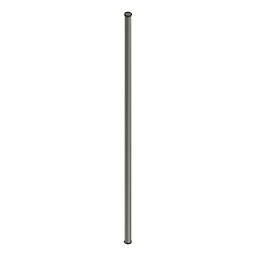
Rainfall sensor mid september v4 (Autodesk Fusion 360 archive; units mm, degrees)
design "graphite rod"
Autodesk Fusion 360 part; units mm, degrees
sketch "Sketch1" plane through (0, 0, 0) normal (0, 0, 1) x (1, 0, 0)
  circle A0 centre (0, 0) radius 1
  dimension "d1" = 2
  constraint coincident A0.centre origin
  measures "d1" diameter of A0
extrude "Extrude1" add sketch "Sketch1" along normal blind 80

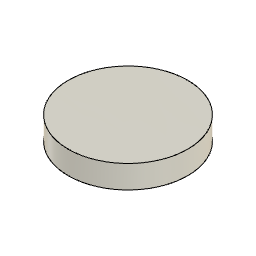
design "PVC_blocker"
Autodesk Fusion 360 part; units mm, degrees
sketch "Sketch1" plane through (0, 0, 0) normal (0, 0, 1) x (1, 0, 0)
  circle A0 centre (0, 0) radius 26
  dimension "d1" = 52
  constraint coincident A0.centre origin
  measures "d1" diameter of A0
extrude "Extrude1" add sketch "Sketch1" along normal blind 10

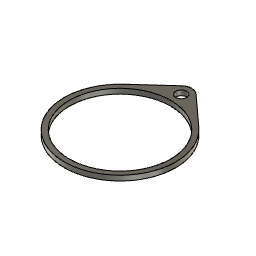
design "External_syphon_holder"
Autodesk Fusion 360 part; units mm, degrees
sketch "Sketch1" plane through (0, 0, 0) normal (0, 0, 1) x (1, 0, 0)
  circle A0 centre (0, 0) radius 30.25
  circle A1 centre (0, 0) radius 33.25
  circle A2 centre (0, 36.5) radius 3.25
  circle A3 centre (0, 36.5) radius 6.25
  line L0 (-22.3742, 24.5959) -> (-4.2057, 41.1233)
  line L1 (22.3742, 24.5959) -> (4.2057, 41.1233)
  dimension "d1" = 60.5
  dimension "d2" = 3
  dimension "d3" = 6.5
  constraint coincident A0.centre A1.centre
  constraint concentric A0 A1
  constraint tangent A1 A2
  constraint concentric A2 A3
  constraint tangent A0 A3
  constraint vertical A0.centre A2.centre
  constraint coincident A1 L0.start
  constraint coincident A3 L0.end
  constraint tangent A3 L0
  constraint coincident A1 L1.start
  constraint coincident A3 L1.end
  constraint tangent A3 L1
  constraint tangent A1 L0
  constraint tangent A1 L1
  measures "d1" diameter of A0
  measures "d2" distance of A0 A1
  measures "d3" diameter of A2
extrude "Extrude1" add sketch "Sketch1" along normal blind 3

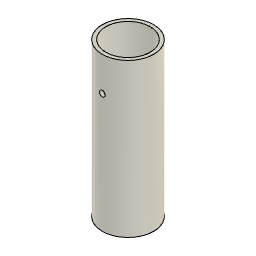
design "PVC 2  D 6  H"
Autodesk Fusion 360 part; units mm, degrees
sketch "Sketch1" plane through (0, 0, 0) normal (0, 0, 1) x (1, 0, 0)
  circle A0 centre (0, 0) radius 30.1625
  circle A1 centre (0, 0) radius 26
  dimension "d1" = 52
  dimension "d2" = 60.325
  constraint coincident A0.centre A1.centre
  measures "d1" diameter of A1
  measures "d2" diameter of A0
extrude "Extrude1" add sketch "Sketch1" along normal blind 180
sketch "Sketch2" plane through (0, 0, 0) normal (0, 1, 0) x (1, 0, 0)
  circle A0 centre (0, -140) radius 3.25
  circle A1 centre (0, -30) radius 2.5
  line L0 (-30.1625, -180) -> (30.1625, -180)
  line L1 (-30.1625, 0) -> (30.1625, 0)
  dimension "d5" = 5
  dimension "d6" = 6.5
  dimension "d7" = 40
  dimension "d8" = 30
  measures "d5" diameter of A1
  measures "d6" diameter of A0
  measures "d7" distance of A0.centre L0
  measures "d8" distance of A1.centre L1
extrude "Extrude2" cut sketch "Sketch2" against normal blind 50 contours A0
extrude "Extrude3" cut sketch "Sketch2" along normal blind 50 contours A1

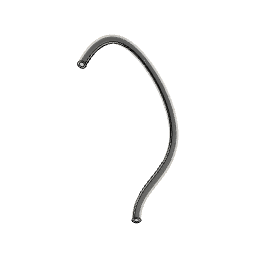
design "syphon v2"
Autodesk Fusion 360 part; units mm, degrees
sketch "Sketch1" plane through (0, 0, 0) normal (0, 0, 1) x (1, 0, 0)
  circle A0 centre (36.5, 0) radius 3.05
  circle A1 centre (36.5, 0) radius 1.8
  dimension "d1" = 6.1
  dimension "d2" = 1.25
  dimension "d3" = 36.5
  constraint concentric A0 A1
  constraint horizontal origin A0.centre
  measures "d1" diameter of A0
  measures "d2" distance of A0 A1
  measures "d3" distance of origin A0.centre
sketch "Sketch2" plane through (0, 0, 0) normal (0, 1, 0) x (1, 0, 0)
  spline S0 degree 5 poles (36, 0) (36, -2.8409) (36.5472, -8.5567) (39.0096, -17.2322) (45.1711, -29.0438) (55.3652, -44.3876) (65.1328, -60.4272) (71.6291, -77.085) (72.709, -93.9676) (67.7291, -110.1794) (57.9485, -124.2901) (45.5412, -134.7685) (32.7553, -140.4361) (21.2769, -140.738) (10.8901, -136.6085) (1.3997, -128.6975) (-5.5417, -119.6353) (-10.404, -111.3808) (-13.4933, -105.2342) (-15, -102) knots 0 0 0 0 0 0 0.066667 0.133333 0.2 0.266667 0.333333 0.4 0.466667 0.533333 0.6 0.666667 0.733333 0.8 0.866667 0.933333 1 1 1 1 1 1
  line L0 (36, 19.394) -> (36, -19.394)
  line L1 (43.5534, -140) -> (8.4466, -140)
  point P0 (71.5, -90)
  point P1 (26, -140)
  point P2 (36.5, 0)
  point P3 (36.5, 0)
  dimension "d4" = 140
  dimension "d5" = 38
  dimension "d6" = 15
  dimension "d7" = 90
  dimension "d8" = 35
  dimension "d15" = 26
  constraint midpoint S0.start L0
  constraint vertical L0
  constraint midpoint P1 L1
  constraint perpendicular L0 L1
  measures "d4" vertical distance of P1 P2
  measures "d5" distance of P1 S0.end
  measures "d6" distance of S0.end origin
  measures "d7" vertical distance of P0 P3
  measures "d8" horizontal distance of P0 P3
  measures "d15" horizontal distance of P1 origin
sweep "Sweep1" add profiles "Sketch1" path "Sketch2" along S0 section 1

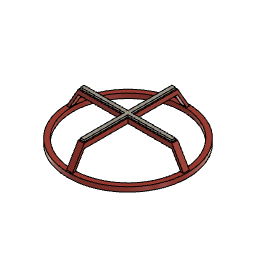
design "PVC metal holder"
Autodesk Fusion 360 part; units mm, degrees
sketch "Sketch1" plane through (0, 0, 0) normal (0, 0, 1) x (1, 0, 0)
  circle A0 centre (0, 0) radius 20
  circle A1 centre (0, 0) radius 25.5
  line L0 (-1.25, 19.9609) -> (-1.25, 1.25)
  line L1 (-1.25, -1.25) -> (-1.25, -19.9609)
  line L2 (-19.9609, 1.25) -> (-1.25, 1.25)
  line L3 (1.25, 1.25) -> (19.9609, 1.25)
  line L4 (1.25, 19.9609) -> (1.25, 1.25)
  line L5 (1.25, -1.25) -> (1.25, -19.9609)
  line L6 (19.9609, -1.25) -> (1.25, -1.25)
  line L7 (-1.25, -1.25) -> (-19.9609, -1.25)
  circle A2 centre (0, 0) radius 23.5
  dimension "d1" = 40
  dimension "d5" = 51
  dimension "d6" = 2.5
  dimension "d7" = 2.5
  dimension "d8" = 2
  constraint coincident A0.centre A1.centre
  constraint coincident A0 L2.start
  constraint coincident A0 L3.end
  constraint horizontal L2
  constraint coincident A0 L6.start
  constraint coincident A0 L7.end
  constraint parallel L2 L6
  constraint coincident A0 L0.start
  constraint coincident A0 L1.end
  constraint perpendicular L0 L2
  constraint coincident A0 L4.start
  constraint coincident A0 L5.end
  constraint perpendicular L4 L6
  constraint coincident L1.start L6
  constraint collinear L0 L1
  constraint collinear L2 L3
  constraint collinear L4 L5
  constraint collinear L6 L7
  constraint equal L2 L3
  constraint equal L2 L7
  measures "d1" diameter of A0
  measures "d5" diameter of A1
  measures "d6" distance of L3 L6
  measures "d7" distance of L0 L4
  measures "d8" distance of A1 A2
extrude "Extrude2" add sketch "Sketch1" along normal blind 2 contours A0 L0 L1 L2 L3 L4 L5 L6 L7
sketch "Sketch3" plane through (0, -1.25, 0) normal (0, -1, 0) x (1, 0, 0)
  line L0 (1.25, 0) -> (19.9609, 0)
  line L1 (19.9609, 0) -> (19.9609, 2)
  line L2 (19.9609, 2) -> (1.25, 2)
  line L3 (1.25, 2) -> (1.25, 0)
  line L4 (24.9609, -8.6603) -> (19.9609, 0)
  line L5 (19.9609, 2) -> (24.9609, -6.6603)
  line L6 (24.9609, -6.6603) -> (24.9609, -8.6603)
  line L7 (25.5, 0) -> (-25.5, 0)
  dimension "d11" = 5
  dimension "d12" = 120
  constraint coincident L0.end L1.start
  constraint coincident L1.end L2.start
  constraint parallel L4 L5
  constraint perpendicular L2 L6
  measures "d11" distance of L1 L6
  measures "d12" angle of L4 L7
extrude "Extrude3" add sketch "Sketch3" against normal up to surface (2.5 mm away) contours L4 L5 L6 L7 | L1 L5 L7
pattern_circular "C-Pattern1" count 4 over 360 about axis through (0, 0, 1.75) along (0, 0, 1) of "Extrude3"
extrude "Extrude4" add sketch "Sketch1" against normal blind 2 from surface at -6.6603 contours A1
sketch "Sketch4" plane through (0, 0, 2) normal (0, 0, 1) x (-1, 0, 0)
  arc A0 (1.25, 19.9609) -> (-1.25, 19.9609) centre (0, 0) ccw
  line L0 (-1.25, 19.9609) -> (-1.25, 1.25)
  line L1 (-1.25, 1.25) -> (-19.9609, 1.25)
  arc A1 (-19.9609, 1.25) -> (-19.9609, -1.25) centre (0, 0) ccw
  line L2 (-19.9609, -1.25) -> (-1.25, -1.25)
  line L3 (-1.25, -1.25) -> (-1.25, -19.9609)
  arc A2 (-1.25, -19.9609) -> (1.25, -19.9609) centre (0, 0) ccw
  line L4 (1.25, -19.9609) -> (1.25, -1.25)
  line L5 (1.25, -1.25) -> (19.9609, -1.25)
  arc A3 (19.9609, -1.25) -> (19.9609, 1.25) centre (0, 0) ccw
  line L6 (19.9609, 1.25) -> (1.25, 1.25)
  line L7 (1.25, 1.25) -> (1.25, 19.9609)
  line L8 (19.4856, 0.75) -> (0.75, 0.75)
  line L9 (0.75, 0.75) -> (0.75, 19.4856)
  arc A4 (0.75, 19.4856) -> (-0.75, 19.4856) centre (0, 0) ccw
  line L10 (-0.75, 19.4856) -> (-0.75, 0.75)
  line L11 (-0.75, 0.75) -> (-19.4856, 0.75)
  arc A5 (-19.4856, 0.75) -> (-19.4856, -0.75) centre (0, 0) ccw
  line L12 (-19.4856, -0.75) -> (-0.75, -0.75)
  line L13 (-0.75, -0.75) -> (-0.75, -19.4856)
  arc A6 (-0.75, -19.4856) -> (0.75, -19.4856) centre (0, 0) ccw
  line L14 (0.75, -19.4856) -> (0.75, -0.75)
  line L15 (0.75, -0.75) -> (19.4856, -0.75)
  arc A7 (19.4856, -0.75) -> (19.4856, 0.75) centre (0, 0) ccw
  dimension "d20" = -0.5
extrude "Extrude5" add sketch "Sketch4" along normal blind 0.75 contours L8 L9 A4 L10 L11 A5 L12 L13 A6 L14 L15 A7

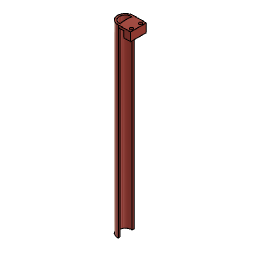
design "PVC_electronics_guide"
Autodesk Fusion 360 part; units mm, degrees
sketch "Sketch1" plane through (0, 0, 0) normal (0, 0, 1) x (1, 0, 0)
  circle A0 centre (0, 0) radius 30.5
  circle A1 centre (0, 0) radius 26.25
  circle A2 centre (0, 0) radius 23.75
  circle A3 centre (-30.5, 0) radius 5
  circle A4 centre (-30.5, 0) radius 6.5
  line L0 (-29.8074, -6.463) -> (-19.8074, -6.463)
  line L1 (-19.8074, -6.463) -> (-19.8074, 6.463)
  line L2 (-19.8074, 6.463) -> (-29.8074, 6.463)
  circle A5 centre (-21.8074, 3.75) radius 1.25
  circle A6 centre (-21.8074, -3.75) radius 1.25
  line L3 (-21.8074, 3.75) -> (-21.8074, -3.75) construction
  point P0 (-21.8074, 0)
  dimension "d1" = 52.5
  dimension "d2" = 61
  dimension "d3" = 2.5
  dimension "d4" = 10
  dimension "d5" = 1.5
  dimension "d6" = 2.5
  dimension "d7" = 2.5
  dimension "d8" = 10
  dimension "d9" = 7.5
  dimension "d10" = 2
  constraint coincident A0.centre A1.centre
  constraint concentric A0 A1
  constraint concentric A0 A2
  constraint coincident A0 A3.centre
  constraint concentric A3 A4
  constraint horizontal A0.centre A3.centre
  constraint horizontal L0
  constraint perpendicular L0 L1
  constraint parallel L0 L2
  constraint coincident A0 L0.start
  constraint coincident A4 L0.start
  constraint coincident A0 L2.end
  constraint coincident A4 L2.end
  constraint vertical A5.centre A6.centre
  constraint coincident A5.centre L3.start
  constraint coincident A6.centre L3.end
  constraint midpoint L3 P0
  constraint horizontal A0.centre P0
  measures "d1" diameter of A1
  measures "d2" diameter of A0
  measures "d3" distance of A1 A2
  measures "d4" diameter of A3
  measures "d5" distance of A3 A4
  measures "d6" diameter of A5
  measures "d7" diameter of A6
  measures "d8" distance of L1 L2.end
  measures "d9" distance of A5.centre A6.centre
  measures "d10" distance of L1 A5.centre
extrude "Extrude1" add sketch "Sketch1" against normal blind 150 contours A0 A3 A4
extrude "Extrude2" add sketch "Sketch1" along normal blind 2 contours A0 A1 A3 A4 | A0 A3 A4 | A1 A4 L2 | A0 A1 A3 A4 | A1 A4 L0 | A0 A1 A3 | A1 A3 A4 | A1 A2 A4 L0 L2 | A1 A3 | A2 L0 L1 L2 picked at (-22.2695, 0)
extrude "Extrude3" add sketch "Sketch1" against normal blind 5 contours A1 A3 A4 | A1 A2 A4 L0 L2 | A1 A3 | A2 L0 L1 L2 picked at (-22.2695, 0)
